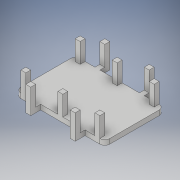
# Autodesk Inventor part: Floor
Saved by Autodesk Inventor 2019 (Build 230136000, 136)
## iProperties
Created: 2018-06-11
Part Number: Floor
Material: Ogólny
Document SubType Name: Modeling
Designer: Kamil
Density: 1 g/cm^3
Appearance: Domyślna
Author: Kamil
Autodesk Inventor part; units mm, degrees
ref_plane "YZ Plane" through (0, 0, 0) normal (1, 0, 0) x (0, 1, 0)
ref_plane "XZ Plane" through (0, 0, 0) normal (0, 1, 0) x (-1, 0, 0)
ref_plane "XY Plane" through (0, 0, 0) normal (0, 0, 1) x (1, 0, 0)
sketch "Szkic1" plane through (0, 0, 0) normal (0, 1, 0) x (-1, 0, 0)
  line L0 (40, -30) -> (-40, -30)
  line L1 (-45, -25) -> (-45, 25)
  line L2 (-40, 30) -> (40, 30)
  line L3 (45, 25) -> (45, -25)
  line L4 (45, -30) -> (-45, 30) construction
  line L5 (-45, -30) -> (45, 30) construction
  arc A0 (45, 25) -> (40, 30) centre (40, 25) ccw
  arc A1 (40, -30) -> (45, -25) centre (40, -25) ccw
  arc A2 (-45, -25) -> (-40, -30) centre (-40, -25) ccw
  arc A3 (-40, 30) -> (-45, 25) centre (-40, 25) ccw
  line L6 (40, 30) -> (35, 30)
  line L7 (35, 30) -> (35, 25)
  line L8 (35, 25) -> (40, 25)
  line L9 (40, 25) -> (40, 30)
  line L10 (25, 30) -> (20, 30)
  line L11 (20, 30) -> (20, 25)
  line L12 (20, 25) -> (25, 25)
  line L13 (25, 25) -> (25, 30)
  line L14 (2.5, 30) -> (-2.5, 30)
  line L15 (-2.5, 30) -> (-2.5, 25)
  line L16 (-2.5, 25) -> (2.5, 25)
  line L17 (2.5, 25) -> (2.5, 30)
  line L18 (-20, 30) -> (-25, 30)
  line L19 (-25, 30) -> (-25, 25)
  line L20 (-25, 25) -> (-20, 25)
  line L21 (-20, 25) -> (-20, 30)
  line L22 (-35, 30) -> (-40, 30)
  line L23 (-40, 30) -> (-40, 25)
  line L24 (-40, 25) -> (-35, 25)
  line L25 (-35, 25) -> (-35, 30)
  line L26 (-40, -25) -> (40, -25)
  line L27 (40, -25) -> (35, -25)
  line L28 (35, -25) -> (35, -30)
  line L29 (35, -30) -> (40, -30)
  line L30 (40, -30) -> (40, -25)
  line L31 (25, -25) -> (20, -25)
  line L32 (20, -25) -> (20, -30)
  line L33 (20, -30) -> (25, -30)
  line L34 (25, -30) -> (25, -25)
  line L35 (2.5, -25) -> (-2.5, -25)
  line L36 (-2.5, -25) -> (-2.5, -30)
  line L37 (-2.5, -30) -> (2.5, -30)
  line L38 (2.5, -30) -> (2.5, -25)
  line L39 (-20, -25) -> (-25, -25)
  line L40 (-25, -25) -> (-25, -30)
  line L41 (-25, -30) -> (-20, -30)
  line L42 (-20, -30) -> (-20, -25)
  line L43 (-35, -25) -> (-40, -25)
  line L44 (-40, -25) -> (-40, -30)
  line L45 (-40, -30) -> (-35, -30)
  line L46 (-35, -30) -> (-35, -25)
  point P0 (0, 0)
  point P1 (40, -30)
  dimension "d0" = 90
  dimension "d1" = 60
  dimension "d2" = 5
  dimension "d3" = 5
  dimension "d4" = 5
  dimension "d5" = 5
  dimension "d6" = 5
  dimension "d7" = 5
  dimension "d8" = 5
  dimension "d9" = 5
  dimension "d10" = 5
  dimension "d11" = 5
  dimension "d12" = 5
  dimension "d13" = 5
  dimension "d14" = 5
  dimension "d15" = 5
  dimension "d16" = 5
  dimension "d17" = 5
  dimension "d18" = 5
  dimension "d19" = 5
  dimension "d20" = 5
  dimension "d21" = 5
  dimension "d22" = 5
  constraints: 94 end point, 22 parallel, 14 point on line, 11 horizontal, 11 perpendicular, 8 point on circle, 8 tangent, 4 centre point, 3 equal radius, 2 midpoint
  measures "d0" distance of L4.end L5.end
  measures "d1" distance of L5.start L4.end
  measures "d2" radius of A0
  measures "d3" distance of L8.end L7.end
  measures "d4" distance of L7.end L6.end
  measures "d5" distance of L12.end L11.end
  measures "d6" distance of L11.end L10.end
  measures "d7" distance of L16.end L15.end
  measures "d8" distance of L15.end L14.end
  measures "d9" distance of L20.end L19.end
  measures "d10" distance of L19.end L18.end
  measures "d11" distance of L24.end L23.end
  measures "d12" distance of L23.end L22.end
  measures "d13" distance of L29.end L28.end
  measures "d14" distance of L28.end L28.start
  measures "d15" distance of L34.start L32.end
  measures "d16" distance of L32.end L32.start
  measures "d17" distance of L38.start L37.start
  measures "d18" distance of L37.start L36.start
  measures "d19" distance of L41.end L40.end
  measures "d20" distance of L40.end L39.end
  measures "d21" distance of L46.start L44.end
  measures "d22" distance of L44.end L43.end
extrude "Wyciągnięcie proste1" add sketch "Szkic1" along normal blind 5 contours L30 L26 L44 A2 L1 A3 L23 L24 L25 L2 L19 L20 L21 L15 L16 L17 L11 L12 L13 L7 L8 L9 A0 L3 A1 | L0 L34 L26 L28 | L0 L38 L26 L32 | L0 L42 L26 L36 | L0 L46 L26 L40
sketch "Szkic2" plane through (0, 0, 0) normal (0, -1, 0) x (1, 0, 0)
  line L0 (-35, 30) -> (-40, 30)
  line L1 (-40, 30) -> (-40, 25)
  line L2 (-40, 25) -> (-35, 25)
  line L3 (-35, 25) -> (-35, 30)
  line L4 (2.5, 30) -> (-2.5, 30)
  line L5 (-2.5, 30) -> (-2.5, 25)
  line L6 (-2.5, 25) -> (2.5, 25)
  line L7 (2.5, 25) -> (2.5, 30)
  line L8 (40, 30) -> (35, 30)
  line L9 (35, 30) -> (35, 25)
  line L10 (35, 25) -> (40, 25)
  line L11 (40, 25) -> (40, 30)
  line L12 (-35, -25) -> (-40, -25)
  line L13 (-40, -25) -> (-40, -30)
  line L14 (-40, -30) -> (-35, -30)
  line L15 (-35, -30) -> (-35, -25)
  line L16 (2.5, -25) -> (-2.5, -25)
  line L17 (-2.5, -25) -> (-2.5, -30)
  line L18 (-2.5, -30) -> (2.5, -30)
  line L19 (2.5, -30) -> (2.5, -25)
  line L20 (40, -25) -> (35, -25)
  line L21 (35, -25) -> (35, -30)
  line L22 (35, -30) -> (40, -30)
  line L23 (40, -30) -> (40, -25)
  point P0 (0, 0)
  dimension "d25" = 5
  dimension "d26" = 5
  dimension "d29" = 5
  dimension "d31" = 5
  dimension "d32" = 5
  dimension "d33" = 5
  dimension "d34" = 5
  dimension "d35" = 5
  dimension "d36" = 5
  dimension "d37" = 5
  constraints: 48 end point, 12 parallel, 6 horizontal, 6 perpendicular
  measures "d25" distance of L2.end L1.end
  measures "d26" distance of L1.end L0.end
  measures "d29" distance of L6.end L5.end
  measures "d31" distance of L10.end L9.end
  measures "d32" distance of L9.end L8.end
  measures "d33" distance of L14.end L13.end
  measures "d34" distance of L13.end L12.end
  measures "d35" distance of L18.end L17.end
  measures "d36" distance of L22.end L21.end
  measures "d37" distance of L21.end L20.end
extrude "Wyciągnięcie proste2" add sketch "Szkic2" against normal blind 25
sketch "Szkic5" plane through (0, 0, 0) normal (0, -1, 0) x (1, 0, 0)
  line L0 (25, 25) -> (20, 25)
  line L1 (20, 25) -> (20, 40)
  line L2 (20, 40) -> (25, 40)
  line L3 (25, 40) -> (25, 25)
  line L4 (-20, 25) -> (-25, 25)
  line L5 (-25, 25) -> (-25, 40)
  line L6 (-25, 40) -> (-20, 40)
  line L7 (-20, 40) -> (-20, 25)
  line L8 (25, -25) -> (20, -25)
  line L9 (20, -25) -> (20, -40)
  line L10 (20, -40) -> (25, -40)
  line L11 (25, -40) -> (25, -25)
  line L12 (-20, -25) -> (-25, -25)
  line L13 (-25, -25) -> (-25, -40)
  line L14 (-25, -40) -> (-20, -40)
  line L15 (-20, -40) -> (-20, -25)
  point P0 (0, 0)
  dimension "d56" = 5
  dimension "d57" = 15
  dimension "d58" = 5
  dimension "d59" = 15
  dimension "d60" = 5
  dimension "d61" = 15
  dimension "d62" = 5
  dimension "d63" = 15
  constraints: 32 end point, 8 parallel, 4 horizontal, 4 perpendicular, 4 point on line
  measures "d56" distance of L1.end L2.end
  measures "d57" distance of L0.end L1.end
  measures "d58" distance of L5.end L6.end
  measures "d59" distance of L4.end L5.end
  measures "d60" distance of L10.end L9.end
  measures "d61" distance of L9.end L8.end
  measures "d62" distance of L14.end L13.end
  measures "d63" distance of L13.end L12.end
extrude "Wyciągnięcie proste5" add sketch "Szkic5" against normal blind 5
sketch "Szkic6" plane through (0, 5, 0) normal (0, 1, 0) x (1, 0, 0)
  line L0 (25, -40) -> (20, -40)
  line L1 (20, -40) -> (20, -35)
  line L2 (20, -35) -> (25, -35)
  line L3 (25, -35) -> (25, -40)
  line L4 (-20, -40) -> (-25, -40)
  line L5 (-25, -40) -> (-25, -35)
  line L6 (-25, -35) -> (-20, -35)
  line L7 (-20, -35) -> (-20, -40)
  line L8 (25, 40) -> (20, 40)
  line L9 (20, 40) -> (20, 35)
  line L10 (20, 35) -> (25, 35)
  line L11 (25, 35) -> (25, 40)
  line L12 (-20, 40) -> (-25, 40)
  line L13 (-25, 40) -> (-25, 35)
  line L14 (-25, 35) -> (-20, 35)
  line L15 (-20, 35) -> (-20, 40)
  point P0 (0, 0)
  dimension "d66" = 5
  dimension "d67" = 5
  dimension "d68" = 5
  dimension "d69" = 5
  dimension "d70" = 5
  dimension "d71" = 5
  dimension "d72" = 5
  dimension "d73" = 5
  constraints: 32 end point, 8 parallel, 4 horizontal, 4 perpendicular, 2 point on line
  measures "d66" distance of L1.end L2.end
  measures "d67" distance of L0.end L1.end
  measures "d68" distance of L5.end L6.end
  measures "d69" distance of L4.end L5.end
  measures "d70" distance of L10.end L9.end
  measures "d71" distance of L9.end L8.end
  measures "d72" distance of L14.end L13.end
  measures "d73" distance of L13.end L12.end
extrude "Wyciągnięcie proste6" add sketch "Szkic6" along normal blind 20
